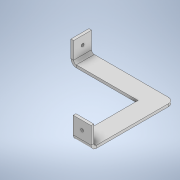
# Autodesk Inventor part: 鋁擠加強肋
Saved by Autodesk Inventor 2021 (Build 250183000, 183)
## iProperties
Created: 2023-02-14
Part Number: 鋁擠加強肋
Material: 一般
Document SubType Name: Sheet Metal
Designer: brian
Density: 1 g/cm^3
Sheet Metal Rule: 預設 mm (_M)
Appearance: 預設
Author: brian
Autodesk Inventor part; units mm, degrees
ref_plane "YZ Plane" through (0, 0, 0) normal (1, 0, 0) x (0, 1, 0)
ref_plane "XZ Plane" through (0, 0, 0) normal (0, 1, 0) x (-1, 0, 0)
ref_plane "XY Plane" through (0, 0, 0) normal (0, 0, 1) x (1, 0, 0)
sketch "草圖1" plane through (0, 0, 0) normal (0, 1, 0) x (-1, 0, 0)
  line L0 (0, 0) -> (0, 92.5)
  line L1 (0, 92.5) -> (20, 92.5)
  line L2 (20, 92.5) -> (20, 20)
  line L3 (20, 20) -> (95, 20)
  line L4 (95, 20) -> (95, 0)
  line L5 (95, 0) -> (0, 0)
  dimension "d0" = 92.5
  dimension "d1" = 95
  dimension "d2" = 20
  dimension "d3" = 20
  measures "d0" distance of L0.start L0.end
  measures "d1" distance of L4.end L0.start
  measures "d2" distance of L0.end L1.end
  measures "d3" distance of L3.end L4.end
extrude "平板1" add sketch "草圖1" along normal blind 3
fillet "轉角外圓角1" radius 6 1 edges at (0, 1.5, 0)
sketch "草圖2" plane through (0, 0, 89.5) normal (0, 0, 1) x (1, 0, 0)
  line L0 (-20, 0) -> (0, 0)
  line L1 (0, 0) -> (0, 25)
  line L2 (0, 25) -> (-20, 25)
  line L3 (-20, 25) -> (-20, 0)
  constraints: 6 end point, 1 horizontal, 1 perpendicular, 1 vertical
edge flange "凸緣1" height 25 angle 90 thickness 3 bend radius 3 thickness toward (0, 0, 1) relief tear relief width 3 relief depth 1.5 corner gap 3 corner form 0 edges at (-10, 3, 92.5) (-95, 3, 10) wall of the first edge with corners at (-20, 0, 89.5) (0, 0, 89.5) (0, 25, 89.5) (-20, 25, 89.5)
bend "折彎1"
corner "轉角1"
sketch "草圖3" plane through (-92, 25, 20) normal (1, 0, 0) x (0, 0, -1)
  line L0 (20, 0) -> (0, 0) projected
  line L1 (20, -19) -> (20, 0) projected
  point P0 (20, -25)
  point P1 (10, -9.5)
  point P2 (10, 0)
  point P3 (20, -9.5)
  constraints: 2 midpoint, 1 horizontal alignment, 1 vertical alignment
hole "孔1" at (-92, 15.5, 10) direction (-1, 0, 0) diameter 3.2 end through all
sketch "草圖4" plane through (0, 25, 89.5) normal (0, 0, -1) x (-1, 0, 0)
  line L0 (20, 0) -> (0, 0) projected
  line L1 (20, -19) -> (20, 0) projected
  point P0 (0, -25)
  point P1 (10, -9.5)
  point P2 (10, 0)
  point P3 (20, -9.5)
  constraints: 2 midpoint, 1 horizontal alignment, 1 vertical alignment
hole "孔2" at (-10, 15.5, 89.5) direction (0, 0, 1) diameter 3.2 end through all
equation "\"d21\" = 厚度"
equation "\"d28\" = 厚度"
equation "\"d4\" = 厚度"
equation "\"d6\" = 折彎離隙寬度"
equation "\"d7\" = 折彎離隙深度"
equation "\"d8\" = 最小剩餘"
equation "\"d9\" = 轉移半徑"
equation "\"d12\" = 折彎半徑"
equation "\"d13\" = 轉角離隙大小"
equation "\"d14\" = 間隙大小"
equation "\"d15\" = Jacobi半徑大小"
equation "\"折彎半徑\" = 厚度"
equation "\"折彎離隙寬度\" = 厚度"
equation "\"折彎離隙深度\" = 0.5 * 厚度"
equation "\"轉角離隙大小\" = 4 * 厚度"
equation "\"最小剩餘\" = 2 * 厚度"
equation "\"轉移半徑\" = 折彎半徑"
equation "\"Jacobi半徑大小\" = 折彎半徑"
equation "\"間隙大小\" = 厚度"
equation "\"厚度\" = 3"
